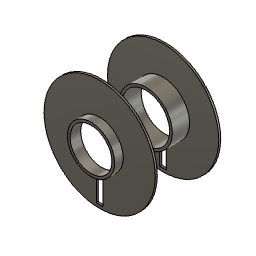
Spool (Autodesk Fusion 360 design; units mm, degrees)
Autodesk Fusion 360 part; units mm, degrees
sketch "SingleSpool" plane through (0, 0, 0) normal (0, 0, 1) x (1, 0, 0)
  circle A0 centre (0, 0) radius 3.2
  circle A1 centre (0, 0) radius 3.6
  circle A2 centre (0, 0) radius 3.65
  circle A3 centre (0, 0) radius 4.05
  circle A4 centre (0, 0) radius 8.5
  circle A5 centre (0, 0) radius 8 construction
  line L0 (0, 0) -> (0, -8.0022) construction
  line L1 (-0.5, -0.0067) -> (-0.5, -7.9844) construction
  line L2 (0.5, 0.0066) -> (0.5, -7.9844) construction
  line L3 (-0.5, -4.019) -> (-0.5, -7.9844)
  line L4 (0.5, -4.019) -> (0.5, -7.9844)
  arc A6 (-0.5, -7.9844) -> (0.5, -7.9844) centre (0, -1.0022) ccw
  point P0 (0.5, 0.0066)
  point P1 (-0.5, -0.0067)
  dimension "d158" = 0.4
  dimension "d159" = 6.4
  dimension "d174" = 0.45
  dimension "d175" = 0.85
  dimension "d185" = 17
  dimension "d187" = 16
  dimension "d188" = 0.5
  dimension "d189" = 0.5
  constraint coincident A0.centre A1.centre
  constraint concentric A0 A5
  constraint vertical L0
  constraint coincident P1 L1.start
  constraint coincident A5 L1.end
  constraint vertical L1
  constraint vertical L2
  constraint coincident P0 L2.start
  constraint coincident A5 L2.end
  constraint coincident A3 L3.start
  constraint coincident L1 L3.start
  constraint coincident L2 L4.start
  constraint coincident A3 L4.start
  constraint coincident L0.end A6
  measures "d159" diameter of A0
  measures "d185" diameter of A4
  measures "d187" diameter of A5
  measures "d188" distance of A0.centre P1
  measures "d189" distance of A0.centre P0
extrude "Extrude29" add sketch "SingleSpool" along normal blind 0.3 contours A3 | A4 makes body 1
extrude "Extrude30" add sketch "SingleSpool" along normal blind 2.65 from surface at 0.3 contours A3 bodies 1
extrude "Extrude32" add sketch "SingleSpool" along normal blind 1.325 from surface at 10 separate body contours A1 makes body 2
extrude "Extrude31" add sketch "SingleSpool" against normal blind 0.3 from surface at 10 contours A1 | A2 | A3 | A4 bodies 2
equation "coilWidth = 2.65 mm"
equation "pusherDiameter = 6 mm"
equation "spacerWidth = 0.3 mm"
equation "d159 = pusherDiameter + 0.4 mm"
equation "d164 = spacerWidth"
equation "d167 = coilWidth"
equation "d177 = -spacerWidth"
equation "d180 = coilWidth / 2"
equation "d187 = d185 - 1 mm"
equation "d189 = d188"
named bodies: "SpoolOuter", "SpoolInner"
